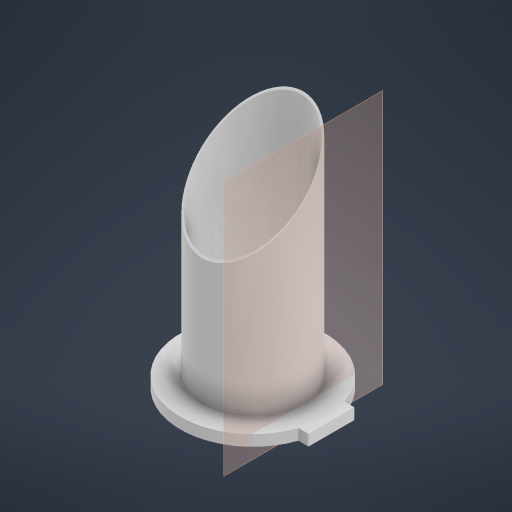
# Autodesk Inventor part: OCAMS
Saved by Autodesk Inventor 2023.2 (Build 272271030, 271C)
## iProperties
Created: 2023-04-10
Part Number: OCAMS
Material: Generic
Document SubType Name: Modeling
Designer: ckeer
Mass: 5150.72 g
Surface Area: 2061.78 cm^2
Volume: 5150.72 cm^3
Density: 1 g/cm^3
Appearance: Default
Author: ckeer
Autodesk Inventor part; units mm, degrees
ref_plane "YZ Plane" through (0, 0, 0) normal (1, 0, 0) x (0, 1, 0)
ref_plane "XZ Plane" through (0, 0, 0) normal (0, 1, 0) x (-1, 0, 0)
ref_plane "XY Plane" through (0, 0, 0) normal (0, 0, 1) x (1, 0, 0)
sketch "Sketch1" plane through (0, 0, 0) normal (0, 1, 0) x (-1, 0, 0)
  circle A0 centre (0, 0) radius 100
  line L0 (-76.20071, 31.896636) -> (-108.814125, 31.896636)
  line L1 (-108.814125, 31.896636) -> (-108.814125, -31.604509)
  line L2 (-108.814125, -31.604509) -> (-76.20071, -31.604509)
  line L3 (-76.20071, -31.604509) -> (-76.20071, 31.896636)
  point P0 (-94.874417, -31.604509)
  point P1 (-94.776604, 31.896636)
  dimension "d0" = 200
  constraints: 8 end point, 2 parallel, 1 centre point, 1 coincident, 1 horizontal, 1 perpendicular
  measures "d0" diameter of A0
sketch "Sketch1 outline for Extrusion1" plane through (0, 0, 0) normal (0, 1, 0) x (-1, 0, 0)
  line L0 (-94.776604, 31.896636) -> (-108.814125, 31.896636)
  line L1 (-108.814125, 31.896636) -> (-108.814125, -31.604509)
  line L2 (-108.814125, -31.604509) -> (-94.874417, -31.604509)
  arc A0 (-94.874417, -31.604509) -> (-94.776604, 31.896636) centre (0, 0) ccw
extrude "Extrusion1" add sketch "Sketch1 outline for Extrusion1" along normal blind 15.24
sketch "Sketch2" plane through (0, 15.24, 0) normal (0, 1, 0) x (-0.0015403, 0, 0.9999988)
  circle A0 centre (0, 0) radius 69.85
  dimension "d3" = 139.7
  constraints: 1 centre point, 1 coincident
  measures "d3" diameter of A0
sketch "Sketch2 outline for Extrusion2" plane through (0, 15.24, 0) normal (0, 1, 0) x (-0.0015403, 0, 0.9999988)
  circle A0 centre (0, 0) radius 69.85
extrude "Extrusion2" add sketch "Sketch2 outline for Extrusion2" along normal blind 304.8
ref_plane "Work Plane1" through (69.85, 15.24, 0) normal (1, 0, 0) x (0, 0, -1)
sketch "Sketch3" plane through (69.85, 15.24, 0) normal (1, 0, 0) x (0, 0, -1)
  line L0 (-69.85, 0) -> (-69.85, 304.8)
  line L1 (69.85, 304.8) -> (-69.85, 304.8)
  line L2 (-69.85, 174.745803) -> (69.85, 304.8)
  line L3 (69.85, 304.8) -> (-69.85, 304.8)
  line L4 (-69.85, 304.8) -> (-69.85, 174.745803)
  point P0 (0, -15.24)
  constraints: 6 end point, 1 collinear, 1 perpendicular, 1 point on line
sketch "Sketch3 outline for Extrusion3" plane through (69.85, 15.24, 0) normal (1, 0, 0) x (0, 0, -1)
  line L0 (-69.85, 174.745803) -> (69.85, 304.8)
  line L1 (-69.85, 304.8) -> (-69.85, 174.745803)
  line L2 (69.85, 304.8) -> (-69.85, 304.8)
extrude "Extrusion3" cut sketch "Sketch3 outline for Extrusion3" against normal through all
shell "Shell1" thickness 2.54 removed faces 1 at (-23.178976, 247.634165, 7.925999)
body "Solid1"
